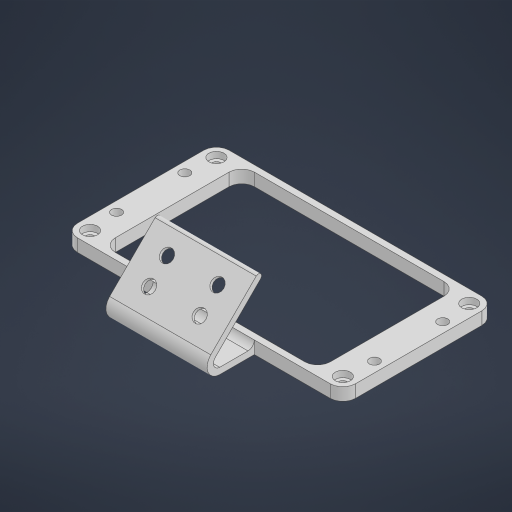
# Autodesk Inventor part: pad
Saved by Autodesk Inventor 2024 (Build 280153000, 153)
## iProperties
Created: 2024-06-08
Part Number: pad
Material: Generic
Document SubType Name: Modeling
Designer: markm
Density: 1 g/cm^3
Appearance: Default
Author: markm
Autodesk Inventor part; units mm, degrees
ref_plane "YZ Plane" through (0, 0, 0) normal (1, 0, 0) x (0, 1, 0)
ref_plane "XZ Plane" through (0, 0, 0) normal (0, 1, 0) x (-1, 0, 0)
ref_plane "XY Plane" through (0, 0, 0) normal (0, 0, 1) x (1, 0, 0)
sketch "Sketch1" plane through (0, 0, 0) normal (0, 1, 0) x (-1, 0, 0)
  line L0 (0, 0) -> (0, 150.5)
  line L1 (47.6822, -16.05) -> (47.6822, -184.7082) construction
  line L2 (47.6822, -184.7082) -> (-45.5409, -184.7082) construction
  line L3 (-45.5409, -184.7082) -> (-45.5409, -16.05) construction
  line L4 (-45.5409, -16.05) -> (47.6822, -16.05) construction
  line L5 (51, 71) -> (51, 72) construction
  line L6 (53, 71) -> (53, 72) construction
  line L7 (49, 72) -> (49, 71) construction
  arc A0 (49, 71) -> (53, 71) centre (51, 71) ccw construction
  arc A1 (53, 72) -> (49, 72) centre (51, 72) ccw construction
  line L8 (0, 85) -> (64.5191, 85) construction
  line L9 (51, 99) -> (51, 98) construction
  line L10 (53, 99) -> (53, 98) construction
  line L11 (49, 98) -> (49, 99) construction
  arc A2 (53, 99) -> (49, 99) centre (51, 99) ccw construction
  arc A3 (49, 98) -> (53, 98) centre (51, 98) ccw construction
  line L12 (50, 115) -> (-55, 115)
  line L13 (-55, 115) -> (-55, 55) construction
  line L14 (-55, 55) -> (50, 55)
  line L15 (55, 60) -> (55, 110)
  circle A4 centre (50, 60) radius 1.6
  circle A5 centre (51, 71.5) radius 2
  circle A6 centre (51, 98.5) radius 2
  line L16 (0, 57.5) -> (37.5, 57.5)
  line L17 (42.5, 62.5) -> (42.5, 107.5)
  line L18 (37.5, 112.5) -> (0, 112.5)
  circle A7 centre (50, 110) radius 1.6
  line L19 (50, 60) -> (50, 110) construction
  arc A8 (50, 55) -> (55, 60) centre (50, 60) ccw
  arc A9 (55, 110) -> (50, 115) centre (50, 110) ccw
  arc A10 (37.5, 57.5) -> (42.5, 62.5) centre (37.5, 62.5) ccw
  arc A11 (42.5, 107.5) -> (37.5, 112.5) centre (37.5, 107.5) ccw
  point P0 (51, 74)
  point P1 (51, 69)
  point P2 (51, 96)
  point P3 (51, 101)
  point P4 (55, 115)
  point P5 (55, 55)
  point P6 (0, 55)
  point P7 (0, 115)
  point P8 (42.5, 57.5)
  point P9 (42.5, 112.5)
  point P10 (0, 113)
  dimension "d9" = 4
  dimension "d10" = 5
  dimension "d12" = 51
  dimension "d22" = 27
  dimension "d29" = 110
  dimension "d31" = 55
  dimension "d85" = 2.5
  dimension "d86" = 42.5
  dimension "d91" = 3.2
  dimension "d92" = 50
  dimension "d99" = 5
  constraints: 36 end point, 18 point on circle, 12 centre point, 12 point on line, 12 tangent, 9 symmetric about line, 5 equal radius, 4 coincident, 3 horizontal, 3 parallel, 3 perpendicular, 3 vertical, 2 midpoint, 8 other
  measures "d9" diameter of A1
  measures "d10" distance of point (51, 74) point (51, 69)
  measures "d12" distance between parallel lines of L0 L5
  measures "d22" distance of point (51, 71.5) A6.centre
  measures "d29" distance of L13.end point (55, 55)
  measures "d31" distance from line of L14 L0.start
  measures "d85" distance between parallel lines of L14 L16
  measures "d86" distance between parallel lines of L0 L17
  measures "d91" diameter of A4
  measures "d92" distance of L19.start L19.end
  measures "d99" radius of A8
extrude "Extrusion1" add sketch "Sketch1" along normal blind 5 contours L16 A10 L17 A11 L18 L0 L12 A9 L15 A8 L14
sketch "Sketch4" plane through (0, 5, 0) normal (0, 1, 0) x (1, 0, 0)
  circle A0 centre (-50, -60) radius 1.6 construction
  circle A1 centre (-50, -60) radius 3
  circle A2 centre (-50, -110) radius 1.6 construction
  circle A3 centre (-50, -110) radius 3
  point P0 (0, 0)
  dimension "d93" = 6
  constraints: 2 centre point, 1 equal radius
  measures "d93" diameter of A1
extrude "Extrusion5" cut sketch "Sketch4" against normal blind 2.5
sketch "Sketch7" plane through (0, 0, 115) normal (1, 0, 0) x (0, 0, -1)
  line L0 (0, 0) -> (2.5, 0) construction
  line L1 (2.5, 0) -> (2.5, 5) construction
  line L2 (0, 5) -> (2.5, 5) construction
  line L3 (0, 0) -> (0, 5) projected
  line L4 (2.5, 0) -> (-25.7843, 0)
  line L5 (-25.7843, 0) -> (2.5, 28.2843)
  line L6 (2.5, 28.2843) -> (2.5, 0)
  line L7 (2.5, 0) -> (2.5, 5) projected
  line L8 (-22.2487, 0) -> (2.5, 24.7487)
  line L9 (0, 5) -> (0, 22.2487)
  line L10 (-23.2843, 2.5) -> (2.5, 2.5)
  line L11 (2.5, 24.7487) -> (0.7322, 26.5165)
  arc A0 (2.5, 24.7487) -> (0.7322, 26.5165) centre (1.6161, 25.6326) ccw
  arc A1 (-17.2487, 8.5355) -> (-13.7132, 0) centre (-13.7132, 5) ccw
  arc A2 (-15.481, 6.7678) -> (-13.7132, 2.5) centre (-13.7132, 5) ccw
  line L12 (-11.6421, 14.1421) -> (-17.2639, 19.7639) construction
  arc A3 (-2.5, 2.5) -> (0, 5) centre (-2.5, 5) ccw
  line L13 (0, 0) -> (0, 5) projected
  point P0 (115, 0)
  point P1 (-19.7487, 2.5)
  point P2 (0, 2.5)
  dimension "d159" = 2.5
  dimension "d160" = 45
  dimension "d161" = 40
  dimension "d184" = 2.5
  dimension "d197" = 5
  constraints: 16 end point, 10 point on line, 8 point on circle, 6 tangent, 4 centre point, 2 midpoint, 2 parallel, 2 perpendicular, 1 collinear, 1 horizontal, 1 vertical
  measures "d159" distance between parallel lines of L8 L5
  measures "d160" angle of L6 L8
  measures "d161" distance of L4.end L5.end
  measures "d184" distance between parallel lines of L4 L10
  measures "d197" radius of A1
extrude "Extrusion15" add sketch "Sketch7" against normal blind 20 contours L4 A1 L10 L3 | L3 L10 L6 L4 | L10 A3 L3 | A1 L8 A2 L10 | L8 A1 L5 L11 | L11 A0 L6 | L6 A0
sketch "Sketch9" plane through (-20, 28.2843, 112.5) normal (0, 0.7071, 0.7071) x (1, 0, 0)
  circle A0 centre (10, -10) radius 2.5
  line L0 (20, -2.5) -> (20, -27.9289) construction
  line L1 (0, -27.9289) -> (0, -2.5) construction
  line L2 (0, -15) -> (20, -15) construction
  circle A1 centre (10, -20) radius 2.5
  line L3 (20, -27.9289) -> (0, -27.9289) construction
  circle A2 centre (10, -10) radius 4.5
  circle A3 centre (10, -10) radius 5 construction
  line L4 (10, -20) -> (10, -10) construction
  line L5 (10, -10) -> (20, -10) construction
  line L6 (10, -20) -> (20, -20) construction
  circle A4 centre (10, -20) radius 4.5
  circle A5 centre (10, -20) radius 5 construction
  line L7 (20, -2.5) -> (0, -2.5) construction
  line L8 (20, 0) -> (0, 0) construction
  point P0 (20, 59.5495)
  dimension "d183" = 5
  dimension "d187" = 9
  dimension "d188" = 10
  dimension "d189" = 10
  dimension "d195" = 2.5
  dimension "d196" = 15
  dimension "d198" = 10
  constraints: 10 end point, 6 centre point, 2 perpendicular, 2 point on line, 1 coincident, 1 parallel, 1 symmetric about line, 1 vertical, 3 other
  measures "d183" diameter of A0
  measures "d187" diameter of A2
  measures "d188" diameter of A3
  measures "d189" distance of L4.start L4.end
  measures "d195" distance between parallel lines of L7 L8
  measures "d196" distance between parallel lines of L2 L8
  measures "d198" distance of L4.end L5.end
extrude "Extrusion16" cut sketch "Sketch9" against normal up to next contours A0 | A1 | A2 | A4
extrude "Extrusion17" add sketch "Sketch9" against normal blind 1.25
mirror "Mirror2" about plane through (0, 0, 0) normal (1, 0, 0)
body "Solid1"
